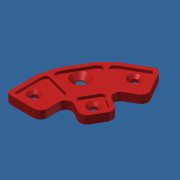
# Autodesk Inventor part: BaseFeet
Saved by Autodesk Inventor 2014 SP2 (Build 180246200, 246)
## iProperties
Created: 2015-02-22
Part Number: BaseFeet
Material: Gummi, Silikon
Document SubType Name: Modeling
Designer: 4ndreas
Density: 1.25 g/cm^3
Appearance: Hellrot
Author: 4ndreas
Autodesk Inventor part; units mm, degrees
ref_plane "YZ Plane" through (0, 0, 0) normal (1, 0, 0) x (0, 1, 0)
ref_plane "XZ Plane" through (0, 0, 0) normal (0, 1, 0) x (-1, 0, 0)
ref_plane "XY Plane" through (0, 0, 0) normal (0, 0, 1) x (1, 0, 0)
sketch "Skizze1" plane through (0, 0, 0) normal (0, 0, 1) x (1, 0, 0)
  arc A0 (-87.287278, 101.151672) -> (-87.483939, 97.817123) centre (-86.287278, 99.419621) ccw
  arc A1 (-85.984849, 96.130127) -> (-87.483939, 97.817123) centre (-90.834591, 93.330127) ccw
  line L0 (-85.984849, 96.130127) -> (-77.984849, 82.273721)
  arc A2 (-80.034591, 74.623978) -> (-77.984849, 82.273721) centre (-82.834591, 79.473721) ccw
  line L1 (-80.034591, 74.623978) -> (-87.443557, 70.34641)
  arc A3 (-87.443557, 70.34641) -> (-87.443557, 62.725387) centre (-85.243557, 66.535898) ccw
  line L2 (-87.443557, 62.725387) -> (-81.953175, 59.555514)
  arc A4 (-79.903433, 51.905771) -> (-81.953175, 59.555514) centre (-84.753175, 54.705771) ccw
  line L3 (-79.903433, 51.905771) -> (-84.903433, 43.245517)
  arc A5 (-92.553175, 41.195775) -> (-84.903433, 43.245517) centre (-89.753175, 46.045517) ccw
  line L4 (-92.553175, 41.195775) -> (-98.043557, 44.365648)
  arc A6 (-98.043557, 44.365648) -> (-104.643557, 40.555136) centre (-100.243557, 40.555136) ccw
  line L5 (-104.643557, 40.555136) -> (-104.643557, 32)
  arc A7 (-110.243557, 26.4) -> (-104.643557, 32) centre (-110.243557, 32) ccw
  line L6 (-110.243557, 26.4) -> (-126.243557, 26.4)
  arc A8 (-128.454083, 26.854752) -> (-126.243557, 26.4) centre (-126.243557, 32) ccw
  arc A9 (-128.454083, 26.854752) -> (-131.243557, 25.017164) centre (-129.243557, 25.017164) ccw
  circle A10 centre (-121.243557, 38.5) radius 2.5
  circle A11 centre (-114.315353, 66) radius 2.5
  circle A12 centre (-93.963756, 85.75) radius 2.5
  circle A13 centre (-91.583302, 52.875644) radius 2.5
  line L7 (-108.923048, 88.660254) -> (-117.975607, 79.660254)
  line L8 (-117.975607, 79.660254) -> (-127.975607, 62.339746)
  line L9 (-127.975607, 62.339746) -> (-131.243557, 50)
  line L10 (-131.243557, 25.017164) -> (-131.243557, 50)
  line L11 (-87.287278, 101.151672) -> (-108.923048, 88.660254)
  constraints: 24 end point, 20 point on circle, 14 centre point, 1 horizontal, 1 parallel, 1 tangent, 1 vertical, 58 other
extrude "Extrusion1" add sketch "Skizze1" along normal blind 6
sketch "Skizze2" plane through (0, 0, 6) normal (0, 0, 1) x (1, 0, 0)
  circle A0 centre (-91.583302, 52.875644) radius 2.5
  circle A1 centre (-93.963756, 85.75) radius 2.5
  circle A2 centre (-114.315353, 66) radius 2.5
  circle A3 centre (-121.243557, 38.5) radius 2.5
  arc A4 (-87.287278, 101.151672) -> (-87.483939, 97.817123) centre (-86.287278, 99.419621) ccw
  line L0 (-87.287278, 101.151672) -> (-108.923048, 88.660254)
  line L1 (-108.923048, 88.660254) -> (-117.975607, 79.660254)
  line L2 (-117.975607, 79.660254) -> (-127.975607, 62.339746)
  line L3 (-127.975607, 62.339746) -> (-131.243557, 50)
  line L4 (-131.243557, 50) -> (-131.243557, 25.017164)
  arc A5 (-128.454083, 26.854752) -> (-131.243557, 25.017164) centre (-129.243557, 25.017164) ccw
  arc A6 (-128.454083, 26.854752) -> (-126.243557, 26.4) centre (-126.243557, 32) ccw
  line L5 (-126.243557, 26.4) -> (-110.243557, 26.4)
  arc A7 (-110.243557, 26.4) -> (-104.643557, 32) centre (-110.243557, 32) ccw
  line L6 (-104.643557, 32) -> (-104.643557, 40.555136)
  arc A8 (-98.043557, 44.365648) -> (-104.643557, 40.555136) centre (-100.243557, 40.555136) ccw
  line L7 (-98.043557, 44.365648) -> (-92.553175, 41.195775)
  arc A9 (-92.553175, 41.195775) -> (-84.903433, 43.245517) centre (-89.753175, 46.045517) ccw
  line L8 (-84.903433, 43.245517) -> (-79.903433, 51.905771)
  arc A10 (-79.903433, 51.905771) -> (-81.953175, 59.555514) centre (-84.753175, 54.705771) ccw
  line L9 (-81.953175, 59.555514) -> (-87.443557, 62.725387)
  arc A11 (-87.443557, 70.34641) -> (-87.443557, 62.725387) centre (-85.243557, 66.535898) ccw
  line L10 (-87.443557, 70.34641) -> (-80.034591, 74.623978)
  arc A12 (-80.034591, 74.623978) -> (-77.984849, 82.273721) centre (-82.834591, 79.473721) ccw
  line L11 (-77.984849, 82.273721) -> (-85.984849, 96.130127)
  arc A13 (-85.984849, 96.130127) -> (-87.483939, 97.817123) centre (-90.834591, 93.330127) ccw
  line L12 (-108.616682, 88.259784) -> (-90.910261, 98.482591)
  arc A14 (-88.300046, 97.936799) -> (-87.783105, 97.416498) centre (-86.287278, 99.419621) ccw
  arc A15 (-86.417862, 95.880127) -> (-87.783105, 97.416498) centre (-90.834591, 93.330127) ccw
  line L13 (-86.417862, 95.880127) -> (-78.417862, 82.023721)
  arc A16 (-80.284591, 75.056991) -> (-78.417862, 82.023721) centre (-82.834591, 79.473721) ccw
  line L14 (-80.284591, 75.056991) -> (-87.693557, 70.779423)
  arc A17 (-87.693557, 70.779423) -> (-87.693557, 62.292374) centre (-85.243557, 66.535898) ccw
  line L15 (-87.693557, 62.292374) -> (-82.203175, 59.122501)
  arc A18 (-80.336446, 52.155771) -> (-82.203175, 59.122501) centre (-84.753175, 54.705771) ccw
  line L16 (-80.336446, 52.155771) -> (-85.336446, 43.495517)
  arc A19 (-92.303175, 41.628788) -> (-85.336446, 43.495517) centre (-89.753175, 46.045517) ccw
  line L17 (-92.303175, 41.628788) -> (-97.793557, 44.798661)
  arc A20 (-97.793557, 44.798661) -> (-105.143557, 40.555136) centre (-100.243557, 40.555136) ccw
  line L18 (-105.143557, 40.555136) -> (-105.143557, 32)
  arc A21 (-110.243557, 26.9) -> (-105.143557, 32) centre (-110.243557, 32) ccw
  line L19 (-110.243557, 26.9) -> (-126.243557, 26.9)
  arc A22 (-128.256714, 27.314149) -> (-126.243557, 26.9) centre (-126.243557, 32) ccw
  arc A23 (-128.256714, 27.314149) -> (-128.965779, 27.501684) centre (-129.243557, 25.017164) ccw
  line L20 (-130.743557, 29.4893) -> (-130.743557, 49.934914)
  line L21 (-130.743557, 49.934914) -> (-127.509311, 62.147395)
  line L22 (-127.509311, 62.147395) -> (-117.575878, 79.352605)
  line L23 (-117.575878, 79.352605) -> (-108.616682, 88.259784)
  arc A24 (-130.743557, 29.4893) -> (-128.965779, 27.501684) centre (-128.743557, 29.4893) ccw
  arc A25 (-88.300046, 97.936799) -> (-90.910261, 98.482591) centre (-89.910261, 96.750541) ccw
  point P0 (0, 0)
  point P1 (-88.769329, 99.718659)
  point P2 (-130.743557, 27.017164)
  dimension "d24" = 2
  dimension "d25" = 0.5
  constraints: 26 point on circle, 24 end point, 12 centre point, 4 tangent, 2 point on line, 1 equal radius, 21 other
  measures "d24" radius of A24
  measures "d25" distance between parallel lines of L12 L0
extrude "Extrusion2" cut sketch "Skizze2" against normal through all contours A4 A13 L11 A12 L10 A11 L9 A10 L8 A9 L7 A8 L6 A7 L5 A6 A5 L4 L3 L2 L1 L0
sketch "Skizze3" plane through (0, 0, 6) normal (0, 0, 1) x (1, 0, 0)
  arc A0 (-97.793557, 44.798661) -> (-105.143557, 40.555136) centre (-100.243557, 40.555136) ccw
  line L0 (-97.793557, 44.798661) -> (-92.303175, 41.628788)
  arc A1 (-92.303175, 41.628788) -> (-85.336446, 43.495517) centre (-89.753175, 46.045517) ccw
  line L1 (-85.336446, 43.495517) -> (-80.336446, 52.155771)
  arc A2 (-80.336446, 52.155771) -> (-82.203175, 59.122501) centre (-84.753175, 54.705771) ccw
  line L2 (-82.203175, 59.122501) -> (-87.693557, 62.292374)
  arc A3 (-87.693557, 70.779423) -> (-87.693557, 62.292374) centre (-85.243557, 66.535898) ccw
  line L3 (-87.693557, 70.779423) -> (-80.284591, 75.056991)
  arc A4 (-80.284591, 75.056991) -> (-78.417862, 82.023721) centre (-82.834591, 79.473721) ccw
  line L4 (-78.417862, 82.023721) -> (-86.417862, 95.880127)
  arc A5 (-86.417862, 95.880127) -> (-87.783105, 97.416498) centre (-90.834591, 93.330127) ccw
  arc A6 (-88.300046, 97.936799) -> (-87.783105, 97.416498) centre (-86.287278, 99.419621) ccw
  line L5 (-90.910261, 98.482591) -> (-108.616682, 88.259784)
  line L6 (-108.616682, 88.259784) -> (-117.575878, 79.352605)
  line L7 (-117.575878, 79.352605) -> (-127.509311, 62.147395)
  line L8 (-127.509311, 62.147395) -> (-130.743557, 49.934914)
  line L9 (-130.743557, 49.934914) -> (-130.743557, 29.4893)
  arc A7 (-128.256714, 27.314149) -> (-128.965779, 27.501684) centre (-129.243557, 25.017164) ccw
  arc A8 (-128.256714, 27.314149) -> (-126.243557, 26.9) centre (-126.243557, 32) ccw
  line L10 (-126.243557, 26.9) -> (-110.243557, 26.9)
  arc A9 (-110.243557, 26.9) -> (-105.143557, 32) centre (-110.243557, 32) ccw
  line L11 (-105.143557, 32) -> (-105.143557, 40.555136)
  circle A10 centre (-91.583302, 52.875644) radius 2.5
  circle A11 centre (-93.963756, 85.75) radius 2.5
  circle A12 centre (-114.315353, 66) radius 2.5
  circle A13 centre (-121.243557, 38.5) radius 2.5
  line L12 (-89.015938, 94.380127) -> (-81.015938, 80.523721)
  arc A14 (-81.784591, 77.655067) -> (-81.015938, 80.523721) centre (-82.834591, 79.473721) ccw
  line L13 (-81.784591, 77.655067) -> (-89.193557, 73.377499)
  arc A15 (-89.193557, 73.377499) -> (-89.193557, 59.694298) centre (-85.243557, 66.535898) ccw
  line L14 (-89.193557, 59.694298) -> (-83.703175, 56.524425)
  arc A16 (-82.934522, 53.655771) -> (-83.703175, 56.524425) centre (-84.753175, 54.705771) ccw
  line L15 (-82.934522, 53.655771) -> (-87.934522, 44.995517)
  arc A17 (-90.803175, 44.226864) -> (-87.934522, 44.995517) centre (-89.753175, 46.045517) ccw
  line L16 (-90.803175, 44.226864) -> (-96.293557, 47.396737)
  arc A18 (-96.293557, 47.396737) -> (-108.143557, 40.555136) centre (-100.243557, 40.555136) ccw
  line L17 (-108.143557, 40.555136) -> (-108.143557, 32)
  arc A19 (-110.243557, 29.9) -> (-108.143557, 32) centre (-110.243557, 32) ccw
  line L18 (-110.243557, 29.9) -> (-126.243557, 29.9)
  arc A20 (-127.072504, 30.070532) -> (-126.243557, 29.9) centre (-126.243557, 32) ccw
  arc A21 (-127.072504, 30.070532) -> (-127.743557, 30.308667) centre (-129.243557, 25.017164) ccw
  line L19 (-127.743557, 30.308667) -> (-127.743557, 49.544399)
  line L20 (-127.743557, 49.544399) -> (-124.711534, 60.993286)
  line L21 (-124.711534, 60.993286) -> (-115.177502, 77.506714)
  line L22 (-115.177502, 77.506714) -> (-106.778486, 85.856966)
  line L23 (-106.778486, 85.856966) -> (-90.119853, 95.474832)
  arc A22 (-90.119853, 95.474832) -> (-89.578097, 95.01275) centre (-86.287278, 99.419621) ccw
  arc A23 (-89.015938, 94.380127) -> (-89.578097, 95.01275) centre (-90.834591, 93.330127) ccw
  circle A24 centre (-114.315353, 66) radius 6.5 construction
  circle A25 centre (-91.583302, 52.875644) radius 6.5 construction
  line L24 (-108.616682, 88.259784) -> (-117.575878, 79.352605)
  line L25 (-117.575878, 79.352605) -> (-127.509311, 62.147395)
  line L26 (-127.509311, 62.147395) -> (-130.743557, 49.934914)
  line L27 (-130.743557, 49.934914) -> (-130.743557, 29.4893)
  arc A26 (-130.743557, 29.4893) -> (-128.965779, 27.501684) centre (-128.743557, 29.4893) ccw
  arc A27 (-128.256714, 27.314149) -> (-128.965779, 27.501684) centre (-129.243557, 25.017164) ccw
  arc A28 (-128.256714, 27.314149) -> (-126.243557, 26.9) centre (-126.243557, 32) ccw
  line L28 (-126.243557, 26.9) -> (-110.243557, 26.9)
  arc A29 (-110.243557, 26.9) -> (-105.143557, 32) centre (-110.243557, 32) ccw
  line L29 (-105.143557, 32) -> (-105.143557, 40.555136)
  arc A30 (-97.793557, 44.798661) -> (-105.143557, 40.555136) centre (-100.243557, 40.555136) ccw
  line L30 (-97.793557, 44.798661) -> (-92.303175, 41.628788)
  arc A31 (-92.303175, 41.628788) -> (-85.336446, 43.495517) centre (-89.753175, 46.045517) ccw
  line L31 (-85.336446, 43.495517) -> (-80.336446, 52.155771)
  arc A32 (-80.336446, 52.155771) -> (-82.203175, 59.122501) centre (-84.753175, 54.705771) ccw
  line L32 (-82.203175, 59.122501) -> (-87.693557, 62.292374)
  arc A33 (-87.693557, 70.779423) -> (-87.693557, 62.292374) centre (-85.243557, 66.535898) ccw
  line L33 (-87.693557, 70.779423) -> (-80.284591, 75.056991)
  arc A34 (-80.284591, 75.056991) -> (-78.417862, 82.023721) centre (-82.834591, 79.473721) ccw
  line L34 (-78.417862, 82.023721) -> (-86.417862, 95.880127)
  arc A35 (-86.417862, 95.880127) -> (-87.783105, 97.416498) centre (-90.834591, 93.330127) ccw
  arc A36 (-88.300046, 97.936799) -> (-87.783105, 97.416498) centre (-86.287278, 99.419621) ccw
  arc A37 (-88.300046, 97.936799) -> (-90.910261, 98.482591) centre (-89.910261, 96.750541) ccw
  line L35 (-90.910261, 98.482591) -> (-108.616682, 88.259784)
  circle A38 centre (-91.583302, 52.875644) radius 2.5
  circle A39 centre (-93.963756, 85.75) radius 2.5
  circle A40 centre (-114.315353, 66) radius 2.5
  circle A41 centre (-121.243557, 38.5) radius 2.5
  point P0 (0, 0)
  dimension "d6" = 13
  constraints: 48 end point, 40 point on circle, 26 centre point, 2 coincident, 1 equal radius, 1 tangent, 21 other
  measures "d6" diameter of A24
extrude "Extrusion3" cut sketch "Skizze3" against normal blind 2 contours L12 A14 L13 A15 L14 A16 L15 A17 L16 A18 L17 A19 L18 A20 A21 L19 L20 L21 L22 L23 A22 A23
hole "Bohrung1" at (-114.315353, 66, 4) direction (0, 0, -1) diameter 6 end through all countersink diameter 13 countersink angle 90
sketch "Skizze6" plane through (0, 0, 4) normal (0, 0, 1) x (1, 0, 0)
  line L0 (-115.177502, 77.506714) -> (-106.778486, 85.856966)
  line L1 (-119.944518, 69.25) -> (-115.177502, 77.506714)
  circle A0 centre (-114.315353, 66) radius 6.5
  line L2 (-127.743557, 49.544399) -> (-124.711534, 60.993286)
  circle A1 centre (-91.583302, 52.875644) radius 2.5
  line L3 (-126.611554, 53.818829) -> (-125.843537, 56.718855)
  line L4 (-125.843537, 56.718855) -> (-106.831502, 51.683876)
  line L5 (-106.831502, 51.683876) -> (-107.599519, 48.78385)
  line L6 (-107.599519, 48.78385) -> (-126.611554, 53.818829)
  line L7 (-109.914251, 82.739407) -> (-112.041738, 80.624272)
  line L8 (-112.041738, 80.624272) -> (-98.175301, 66.676857)
  line L9 (-98.175301, 66.676857) -> (-96.047813, 68.791992)
  line L10 (-96.047813, 68.791992) -> (-109.914251, 82.739407)
  line L11 (-100.216762, 68.73024) -> (-97.618686, 67.23024)
  line L12 (-97.618686, 67.23024) -> (-107.032438, 50.925142)
  line L13 (-107.032438, 50.925142) -> (-109.630515, 52.425142)
  line L14 (-109.630515, 52.425142) -> (-100.216762, 68.73024)
  line L15 (-108.788035, 50.631616) -> (-106.264914, 52.254533)
  line L16 (-106.264914, 52.254533) -> (-101.830536, 45.36048)
  line L17 (-101.830536, 45.36048) -> (-104.353657, 43.737563)
  line L18 (-104.353657, 43.737563) -> (-108.788035, 50.631616)
  line L19 (-98.242283, 68.897394) -> (-98.38621, 65.900848)
  line L20 (-98.38621, 65.900848) -> (-90.198596, 65.507591)
  line L21 (-90.198596, 65.507591) -> (-90.054669, 68.504136)
  line L22 (-90.054669, 68.504136) -> (-98.242283, 68.897394)
  line L23 (-114.315353, 66) -> (-91.583302, 52.875644) construction
  arc A2 (-87.693557, 70.779423) -> (-87.693557, 62.292374) centre (-85.243557, 66.535898) ccw construction
  line L24 (-89.015938, 94.380127) -> (-81.015938, 80.523721)
  arc A3 (-89.015938, 94.380127) -> (-89.578097, 95.01275) centre (-90.834591, 93.330127) ccw
  arc A4 (-90.119853, 95.474832) -> (-89.578097, 95.01275) centre (-86.287278, 99.419621) ccw
  line L25 (-106.778486, 85.856966) -> (-90.119853, 95.474832)
  line L26 (-115.177502, 77.506714) -> (-106.778486, 85.856966)
  line L27 (-119.944518, 69.25) -> (-115.177502, 77.506714)
  circle A5 centre (-114.315353, 66) radius 6.5
  line L28 (-124.711534, 60.993286) -> (-119.944518, 69.25)
  line L29 (-127.743557, 49.544399) -> (-124.711534, 60.993286)
  line L30 (-127.743557, 30.308667) -> (-127.743557, 49.544399)
  arc A6 (-127.072504, 30.070532) -> (-127.743557, 30.308667) centre (-129.243557, 25.017164) ccw
  arc A7 (-127.072504, 30.070532) -> (-126.243557, 29.9) centre (-126.243557, 32) ccw
  line L31 (-110.243557, 29.9) -> (-126.243557, 29.9)
  arc A8 (-110.243557, 29.9) -> (-108.143557, 32) centre (-110.243557, 32) ccw
  line L32 (-108.143557, 40.555136) -> (-108.143557, 32)
  arc A9 (-96.293557, 47.396737) -> (-108.143557, 40.555136) centre (-100.243557, 40.555136) ccw
  line L33 (-90.803175, 44.226864) -> (-96.293557, 47.396737)
  arc A10 (-90.803175, 44.226864) -> (-87.934522, 44.995517) centre (-89.753175, 46.045517) ccw
  line L34 (-82.934522, 53.655771) -> (-87.934522, 44.995517)
  arc A11 (-82.934522, 53.655771) -> (-83.703175, 56.524425) centre (-84.753175, 54.705771) ccw
  line L35 (-89.193557, 59.694298) -> (-83.703175, 56.524425)
  arc A12 (-89.193557, 73.377499) -> (-89.193557, 59.694298) centre (-85.243557, 66.535898) ccw
  line L36 (-81.784591, 77.655067) -> (-89.193557, 73.377499)
  arc A13 (-81.784591, 77.655067) -> (-81.015938, 80.523721) centre (-82.834591, 79.473721) ccw
  circle A14 centre (-91.583302, 52.875644) radius 2.5
  circle A15 centre (-93.963756, 85.75) radius 2.5
  circle A16 centre (-121.243557, 38.5) radius 2.5
  point P0 (0, 0)
  point P1 (-126.227545, 55.268842)
  point P2 (-110.977994, 81.68184)
  dimension "d20" = 3
  constraints: 48 end point, 11 parallel, 7 point on line, 6 equal length, 6 perpendicular, 4 midpoint, 2 centre point, 2 collinear, 2 point on circle, 1 tangent, 6 other
  measures "d20" distance between parallel lines of L12 L14
sketch "Skizze6 outline for Extrusion4" plane through (0, 0, 4) normal (0, 0, 1) x (1, 0, 0)
  line L0 (-106.264914, 52.254533) -> (-98.38621, 65.900848)
  line L1 (-98.38621, 65.900848) -> (-90.198596, 65.507591)
  line L2 (-90.198596, 65.507591) -> (-90.054669, 68.504136)
  line L3 (-90.054669, 68.504136) -> (-96.047813, 68.791992)
  line L4 (-96.047813, 68.791992) -> (-109.914251, 82.739407)
  line L5 (-109.914251, 82.739407) -> (-112.041738, 80.624272)
  line L6 (-112.041738, 80.624272) -> (-100.216762, 68.73024)
  line L7 (-100.216762, 68.73024) -> (-109.630515, 52.425142)
  line L8 (-109.630515, 52.425142) -> (-125.843537, 56.718855)
  line L9 (-125.843537, 56.718855) -> (-126.611554, 53.818829)
  line L10 (-126.611554, 53.818829) -> (-107.599519, 48.78385)
  line L11 (-104.353657, 43.737563) -> (-107.599519, 48.78385)
  line L12 (-101.830536, 45.36048) -> (-104.353657, 43.737563)
  line L13 (-106.264914, 52.254533) -> (-101.830536, 45.36048)
extrude "Extrusion4" add sketch "Skizze6 outline for Extrusion4" along normal up to surface (2 mm away)
fillet "Rundung1" radius 2 14 edges at (-126.6116, 53.8188, 5) (-125.8435, 56.7189, 5) (-106.2649, 52.2545, 5) (-103.3983, 47.7979, 5) (-109.6305, 52.4251, 5) (-105.8722, 46.0984, 5) (-107.5995, 48.7839, 5) (-100.2168, 68.7302, 5) (-112.0417, 80.6243, 5) (-96.0478, 68.792, 5) (-92.8585, 68.6388, 5) (-93.0933, 65.6466, 5) (-98.3862, 65.9008, 5) (-109.9143, 82.7394, 5)
sketch "Skizze7" plane through (0, 0, 4) normal (0, 0, 1) x (1, 0, 0)
  arc A0 (-104.235787, 49.099884) -> (-102.087009, 48.237042) centre (-102.553706, 50.181829) ccw
  line L0 (-82.934522, 53.655771) -> (-87.934522, 44.995517)
  arc A1 (-92.818009, 64.291422) -> (-94.639641, 65.720898) centre (-94.735592, 63.723201) ccw
  circle A2 centre (-91.583302, 52.875644) radius 2.5
  circle A3 centre (-91.583302, 52.875644) radius 7.1 construction
  arc A4 (-97.16801, 65.842337) -> (-98.996012, 64.84464) centre (-97.263961, 63.84464) ccw
  line L1 (-98.996012, 64.84464) -> (-105.655112, 53.310741)
  arc A5 (-105.655112, 53.310741) -> (-105.605142, 51.228797) centre (-103.923061, 52.310741) ccw
  line L2 (-105.605142, 51.228797) -> (-104.235787, 49.099884)
  arc A6 (-104.235787, 49.099884) -> (-102.087009, 48.237042) centre (-102.553706, 50.181829) ccw
  arc A7 (-96.293557, 47.396737) -> (-102.087009, 48.237042) centre (-100.243557, 40.555136) ccw
  line L3 (-90.803175, 44.226864) -> (-96.293557, 47.396737)
  arc A8 (-90.803175, 44.226864) -> (-87.934522, 44.995517) centre (-89.753175, 46.045517) ccw
  line L4 (-82.934522, 53.655771) -> (-87.934522, 44.995517)
  arc A9 (-82.934522, 53.655771) -> (-83.703175, 56.524425) centre (-84.753175, 54.705771) ccw
  line L5 (-89.193557, 59.694298) -> (-83.703175, 56.524425)
  arc A10 (-92.818009, 64.291422) -> (-89.193557, 59.694298) centre (-85.243557, 66.535898) ccw
  arc A11 (-92.818009, 64.291422) -> (-94.639641, 65.720898) centre (-94.735592, 63.723201) ccw
  line L6 (-94.639641, 65.720898) -> (-97.16801, 65.842337)
  circle A12 centre (-91.583302, 52.875644) radius 2.5
  line L7 (-102.491086, 48.182809) -> (-92.97308, 64.668479)
  point P0 (0, 0)
  constraints: 4 point on circle, 2 end point, 2 tangent, 1 centre point, 1 coincident, 1 parallel
extrude "Extrusion5" add sketch "Skizze7" along normal up to surface (2 mm away) contours L2 A5 L1 A4 L6 A1 L7 A0
sketch "Skizze8" plane through (0, 0, 6) normal (0, 0, 1) x (1, 0, 0)
  arc A0 (-92.818009, 64.291422) -> (-92.97308, 64.668479) centre (-94.735592, 63.723201) ccw
  arc A1 (-92.818009, 64.291422) -> (-89.193557, 59.694298) centre (-85.243557, 66.535898) ccw
  arc A2 (-96.293557, 47.396737) -> (-102.087009, 48.237042) centre (-100.243557, 40.555136) ccw
  arc A3 (-102.491086, 48.182809) -> (-102.087009, 48.237042) centre (-102.553706, 50.181829) ccw
  line L0 (-92.97308, 64.668479) -> (-102.491086, 48.182809)
  arc A4 (-100.603143, 51.452822) -> (-99.109575, 48.373326) centre (-98.812835, 50.419187) ccw
  arc A5 (-91.447317, 61.644747) -> (-94.861022, 61.398467) centre (-93.070715, 60.364832) ccw
  point P0 (0, 0)
  dimension "d9" = 13
  dimension "d10" = 6
  constraints: 6 point on circle, 4 tangent, 2 centre point, 2 point on line
extrude "Extrusion6" add sketch "Skizze8" against normal up to surface (2 mm away)
chamfer "Fase1" distance 2 angle 45 3 edges at (-123.7436, 38.5, 4) (-94.0833, 52.8756, 4) (-96.4638, 85.75, 4)
